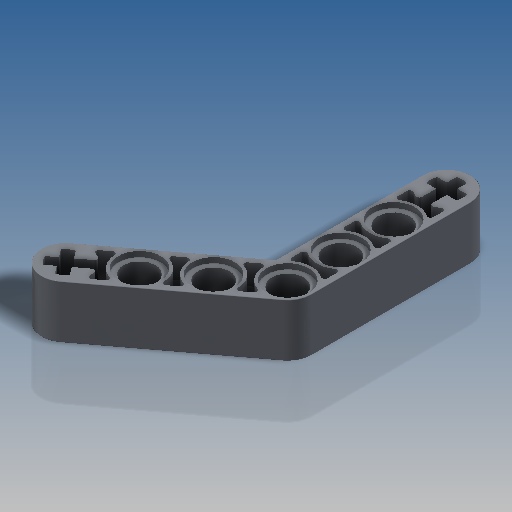
# Autodesk Inventor part: 32348-LtBluishGray
Saved by Autodesk Inventor 2019.4 (Build 234330000, 330)
## iProperties
Created: 2012-03-21
Part Number: 32348-LtBluishGray
Document SubType Name: Modeling
Designer: D. Kohfeld
Density: 1.06 g/cm^3
Material: ABS Plastic
Appearance: LtBluishGray
Mass: 1.80293 g
Surface Area: 29.7146 cm^2
Volume: 1.70088 cm^3
Author: D. Kohfeld
Autodesk Inventor part; units mm, degrees
ref_plane "YZ Plane" through (0, 0, 0) normal (1, 0, 0) x (0, 1, 0)
ref_plane "XZ Plane" through (0, 0, 0) normal (0, 1, 0) x (-1, 0, 0)
ref_plane "XY Plane" through (0, 0, 0) normal (0, 0, 1) x (1, 0, 0)
sketch "Sketch1" plane through (0, 0, 0) normal (0, 0, 1) x (1, 0, 0)
  line L0 (-3.6, 24) -> (-3.6, 0)
  arc A0 (3.6, 24) -> (-3.6, 24) centre (0, 24) ccw
  circle A1 centre (0, 24) radius 3.2 construction
  circle A2 centre (0, 24) radius 2.4 construction
  line L1 (2.7, 21.6188) -> (2.7, 18.3812)
  line L2 (-2.7, 21.6188) -> (-2.7, 18.3812)
  arc A3 (-2.7, 21.6188) -> (2.7, 21.6188) centre (0, 24) ccw
  arc A4 (2.7, 18.3812) -> (-2.7, 18.3812) centre (0, 16) ccw
  circle A5 centre (0, 16) radius 3.2
  circle A6 centre (0, 16) radius 2.4
  line L3 (-0.8, 20.49) -> (-0.8, 23.2)
  line L4 (-0.8, 23.2) -> (-2.2627, 23.2)
  line L5 (-2.2627, 24.8) -> (-0.8, 24.8)
  line L6 (-0.8, 24.8) -> (-0.8, 26.2627)
  line L7 (0.8, 26.2627) -> (0.8, 24.8)
  line L8 (0.8, 24.8) -> (2.2627, 24.8)
  line L9 (2.2627, 23.2) -> (0.8, 23.2)
  line L10 (0.8, 23.2) -> (0.8, 20.49)
  arc A7 (-2.2627, 24.8) -> (-2.2627, 23.2) centre (0, 24) ccw
  arc A8 (0.8, 26.2627) -> (-0.8, 26.2627) centre (0, 24) ccw
  arc A9 (2.2627, 23.2) -> (2.2627, 24.8) centre (0, 24) ccw
  line L11 (3.6, 0) -> (3.6, 24)
  line L12 (2.7, 13.6188) -> (2.7, 10.3812)
  line L13 (-2.7, 13.6188) -> (-2.7, 10.3812)
  arc A10 (-2.7, 13.6188) -> (2.7, 13.6188) centre (0, 16) ccw
  arc A11 (2.7, 10.3812) -> (-2.7, 10.3812) centre (0, 8) ccw
  circle A12 centre (0, 8) radius 3.2
  circle A13 centre (0, 8) radius 2.4
  line L14 (2.7, 5.6188) -> (2.7, 2.3812)
  line L15 (-2.7, 5.6188) -> (-2.7, 2.3812)
  arc A14 (-2.7, 5.6188) -> (2.7, 5.6188) centre (0, 8) ccw
  arc A15 (2.7, 2.3812) -> (-2.7, 2.3812) centre (0, 0) ccw
  circle A16 centre (0, 0) radius 3.2
  circle A17 centre (0, 0) radius 2.4
  arc A18 (-3.6, 0) -> (3.6, 0) centre (0, 0) ccw
  point P0 (-0.8, 12.49)
  point P1 (0.8, 12.49)
  point P2 (-0.8, 4.49)
  point P3 (0.8, 4.49)
  dimension "d32" = 7.2
  dimension "d49" = 6.4
  dimension "d50" = 4.8
  dimension "d51" = 8
  dimension "d52" = 0.9
  dimension "d62" = 1.6
  dimension "d65" = 8
  constraints: 34 point on circle, 32 end point, 19 centre point, 10 coincident, 7 equal radius, 6 equal length, 4 parallel, 4 perpendicular, 4 vertical, 3 tangent, 3 vertical alignment, 2 horizontal alignment, 1 concentric, 32 other
  measures "d32" diameter of A0
  measures "d49" diameter of A1
  measures "d50" diameter of A2
  measures "d51" distance of A0.centre A4.centre
  measures "d52" distance between parallel lines of L0 L2
  measures "d62" distance between parallel lines of L10 L3
  measures "d65" distance of A6.centre A13.centre
extrude "Extrusion1" add sketch "Sketch1" along normal mid plane 8 contours A0 L11 A18 L0 | A5 | L12 A11 L13 A10 | A12 | L14 A15 L15 A14 | A16
sketch "Sketch6" plane through (0, 0, 4) normal (0, 0, 1) x (1, 0, 0)
  circle A0 centre (0, 24) radius 3.2 projected
  line L0 (2.7, 21.6188) -> (2.7, 18.3812) projected
  arc A1 (-2.7, 21.6188) -> (2.7, 21.6188) centre (0, 24) ccw projected
  arc A2 (2.7, 18.3812) -> (-2.7, 18.3812) centre (0, 16) ccw projected
  line L1 (-2.7, 21.6188) -> (-2.7, 18.3812) projected
  arc A3 (-2.8, 21.5813) -> (2.8, 21.5813) centre (0, 24) ccw projected
  arc A4 (2.8, 18.4187) -> (-2.8, 18.4187) centre (0, 16) ccw projected
  line L2 (2.8, 21.5813) -> (2.8, 18.4187) projected
  line L3 (-2.8, 21.5813) -> (-2.8, 18.4187) projected
  circle A5 centre (0, 16) radius 3.2 projected
  circle A6 centre (0, 16) radius 3.1 projected
  line L4 (2.7, 13.6188) -> (2.7, 10.3812) projected
  arc A7 (2.7, 10.3812) -> (-2.7, 10.3812) centre (0, 8) ccw projected
  arc A8 (-2.7, 13.6188) -> (2.7, 13.6188) centre (0, 16) ccw projected
  line L5 (-2.7, 13.6188) -> (-2.7, 10.3812) projected
  line L6 (3.6, 24) -> (3.6, 0) projected
  line L7 (3.6, 0) -> (3.6, 24) projected
  circle A9 centre (0, 8) radius 3.2 projected
  line L8 (2.7, 5.6188) -> (2.7, 2.3812) projected
  arc A10 (-2.7, 5.6188) -> (2.7, 5.6188) centre (0, 8) ccw projected
  arc A11 (2.7, 2.3812) -> (-2.7, 2.3812) centre (0, 0) ccw projected
  line L9 (-2.7, 5.6188) -> (-2.7, 2.3812) projected
  circle A12 centre (0, 0) radius 3.2 projected
extrude "Extrusion7" cut sketch "Sketch6" against normal blind 0.8 contours A5 | A6 | A9 | A12
extrude "Extrusion8" cut sketch "Sketch6" against normal blind 3.1 contours L0 A3 L1 A1 | L0 A4 L1 A3 | L0 A2 L1 A4 | L4 A7 L5 A8 | L8 A11 L9 A10
mirror "Mirror1" about plane through (0, 0, 0) normal (0, 0, 1) of "Extrusion7", "Extrusion8"
pattern_circular "Circular Pattern1" count 2 over 126.87 about axis through (0, 0, -10) along (0, 0, 1) of "Extrusion7", "Extrusion8", "Mirror1", "Extrusion1"
fillet "Fillet2" radius 0.4 44 edges at (-2.7, 5.6188, 2.45) (2.7, 2.3812, 2.45) (2.7, 5.6188, 2.45) (2.7, 10.3812, 2.45) (2.7, 13.6188, 2.45) (-2.7, 10.3812, 2.45) (-2.7, 13.6188, 2.45) (-2.7, 18.3812, 0) (-2.7, 21.6188, 0) (2.7, 18.3812, 0) (2.7, 21.6188, 0) (0.8, 20.49, 0) (-0.8, 20.49, 0) (2.7, 2.3812, -2.45) (2.7, 5.6188, -2.45) (-2.7, 5.6188, -2.45) (-2.7, 10.3812, -2.45) (-2.7, 13.6188, -2.45) (2.7, 13.6188, -2.45) (2.7, 10.3812, -2.45) (-16.872, -11.654, 0) (-15.912, -12.934, 0) (-15.675, -15.1313, 0) (-18.915, -10.8113, 0) (-16.3249, -8.8687, 0) (-13.0849, -13.1887, 0) (-9.275, -10.3313, 2.45) (-6.6849, -8.3887, 2.45) (-9.275, -10.3313, -2.45) (-6.6849, -8.3887, -2.45) (-2.875, -5.5313, 2.45) (-2.875, -5.5313, -2.45) (-0.2849, -3.5887, 2.45) (-0.2849, -3.5887, -2.45) (-6.1151, -1.2113, 2.45) (-3.5249, 0.7313, 2.45) (-12.515, -6.0113, 2.45) (-9.9249, -4.0687, 2.45) (-2.7, 2.475, 2.45) (-2.7, 2.475, -2.45) (-3.5249, 0.7313, -2.45) (-6.1151, -1.2113, -2.45) (-9.9249, -4.0687, -2.45) (-12.515, -6.0113, -2.45)
fillet "Fillet2" radius 0.1 14 edges at (-3.6, 12.9, 4) (0, 27.6, 4) (3.6, 12, 4) (3.2199, -1.61, 4) (0, 27.6, -4) (-3.6, 12.9, -4) (3.2199, -1.61, -4) (3.6, 12, -4) (-22.08, -16.56, -4) (-7.44, -10.08, -4) (-12.48, -4.86, -4) (-22.08, -16.56, 4) (-12.48, -4.86, 4) (-7.44, -10.08, 4)
equation "\"lf\" = 0.1"
equation "\"tf\" = 0.4"
body "Solid1"
